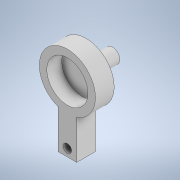
# Autodesk Inventor part: Motorshaft
Saved by Autodesk Inventor 2021 (Build 250183000, 183)
## iProperties
Created: 2021-03-16
Part Number: Motorshaft
Material: Generic
Document SubType Name: Modeling
Designer: Olivi
Density: 1 g/cm^3
Appearance: Default
Author: Olivi
Autodesk Inventor part; units mm, degrees
ref_plane "YZ Plane" through (0, 0, 0) normal (1, 0, 0) x (0, 1, 0)
ref_plane "XZ Plane" through (0, 0, 0) normal (0, 1, 0) x (-1, 0, 0)
ref_plane "XY Plane" through (0, 0, 0) normal (0, 0, 1) x (1, 0, 0)
sketch "Sketch1" plane through (0, 0, 0) normal (0, 0, 1) x (1, 0, 0)
  circle A0 centre (0, 0) radius 3.85
  dimension "d0" = 7.7
  constraints: 1 centre point, 1 coincident
  measures "d0" diameter of A0
extrude "Extrusion1" add sketch "Sketch1" along normal blind 10.2
sketch "Sketch2" plane through (0, 0, 10.2) normal (0, 0, 1) x (1, 0, 0)
  circle A0 centre (0, 0) radius 4
  dimension "d3" = 8
  constraints: 1 centre point, 1 coincident
  measures "d3" diameter of A0
extrude "Extrusion2" add sketch "Sketch2" along normal blind 4 draft 60
sketch "Sketch3" plane through (0, 0, 14.2) normal (0, 0, 1) x (1, 0, 0)
  circle A0 centre (0, 0) radius 15
  dimension "d6" = 30
  constraints: 1 centre point, 1 coincident
  measures "d6" diameter of A0
extrude "Extrusion3" add sketch "Sketch3" along normal blind 10
sketch "Sketch5" plane through (0, 0, 24.2) normal (0, 0, 1) x (1, 0, 0)
  circle A0 centre (0, 0) radius 11
  dimension "d11" = 22
  constraints: 1 centre point, 1 coincident
  measures "d11" diameter of A0
extrude "Extrusion5" cut sketch "Sketch5" against normal blind 8
sketch "Sketch6" plane through (0, 0, 0) normal (0, 0, -1) x (-1, 0, 0)
  circle A0 centre (0, 0) radius 2.55
  dimension "d14" = 5.1
  constraints: 1 centre point, 1 coincident
  measures "d14" diameter of A0
extrude "Extrusion6" cut sketch "Sketch6" against normal blind 1.8
sketch "Sketch7" plane through (0, 0, 1.8) normal (0, 0, -1) x (-1, 0, 0)
  point P0 (0, 0)
sketch "Sketch8" plane through (0, 0, 1.8) normal (0, 0, -1) x (-1, 0, 0)
  line L0 (-1.55, 2.0667) -> (1.55, 2.0667)
  line L1 (1.55, 2.0667) -> (1.55, -2.0667)
  line L2 (1.55, -2.0667) -> (-1.55, -2.0667)
  line L3 (-1.55, -2.0667) -> (-1.55, 2.0667)
  line L4 (-1.55, 2.0667) -> (1.55, -2.0667) construction
  line L5 (1.55, 2.0667) -> (-1.55, -2.0667) construction
  circle A0 centre (0, 0) radius 2.5833
  arc A1 (1.55, 2.0667) -> (-1.55, 2.0667) centre (0, 0) ccw
  arc A2 (-1.55, -2.0667) -> (1.55, -2.0667) centre (0, 0) ccw
  arc A3 (1.55, 2.0667) -> (-1.55, 2.0667) centre (0, 0.6019) ccw
  arc A4 (-1.55, -2.0667) -> (1.55, -2.0667) centre (0, -0.6159) ccw
  dimension "d17" = 3.1
  constraints: 12 end point, 8 point on circle, 4 centre point, 2 midpoint, 2 parallel, 1 coincident, 1 horizontal, 1 perpendicular, 3 other
  measures "d17" distance of L1.end L2.end
extrude "Extrusion7" cut sketch "Sketch8" against normal blind 8 contours A0 L0 | L0 L1 L2 L3 | L2 A0
sketch "Sketch9" plane through (0, 0, 14.2) normal (0, 0, -1) x (-1, 0, 0)
  line L0 (-5, -12) -> (5, -12)
  line L1 (5, -12) -> (5, -35)
  line L2 (5, -35) -> (-5, -35)
  line L3 (-5, -35) -> (-5, -12)
  circle A0 centre (0, 0) radius 15 projected
  point P0 (0, -15)
  dimension "d25" = 20
  dimension "d30" = 5
  dimension "d31" = 5
  dimension "d32" = 3
  constraints: 8 end point, 2 parallel, 1 horizontal, 1 perpendicular, 1 vertical alignment, 1 other
  measures "d25" distance from line of point (0, -15) L2
  measures "d30" distance from line of L3 point (0, -15)
  measures "d31" distance from line of L1 point (0, -15)
  measures "d32" distance from line of L0 point (0, -15)
extrude "Extrusion8" add sketch "Sketch9" against normal blind 10 contours L0 L1 A0 L3 | A0 L1 L2 L3 picked at (0.5652, -12.968)
sketch "Sketch10" plane through (0, 0, 14.2) normal (0, 0, -1) x (-1, 0, 0)
  circle A0 centre (0, -31) radius 2.25
  line L0 (-5, -35) -> (5, -35) projected
  point P0 (0, 0)
  dimension "d33" = 4.5
  dimension "d34" = 4
  constraints: 1 centre point
  measures "d33" diameter of A0
  measures "d34" distance from line of L0 A0.centre
extrude "Extrusion9" cut sketch "Sketch10" against normal through all
body "Solid1"
